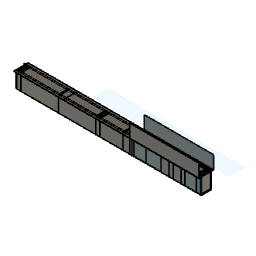
Final Bridge Assembly (Autodesk Fusion 360 design; units mm, degrees)
Autodesk Fusion 360 part; units mm, degrees
sketch "Sketch1" plane through (0, 0, 0) normal (0, 0, 1) x (1, 0, 0) in component "1: Left Top Flange "
  line L0 (20, 60) -> (364, 60)
  line L1 (364, 60) -> (364, -40)
  line L2 (364, -40) -> (20, -40)
  line L3 (20, -40) -> (20, 60)
  dimension "d1" = 344
  dimension "d2" = 100
  constraint horizontal L0
  constraint vertical L1
  constraint horizontal L2
  constraint vertical L3
  measures "d1" distance of L0.start L0.end
  measures "d2" distance of L0.start L2.end
extrude "Extrude1" add sketch "Sketch1" along normal blind 1.27 makes body 1 in component "1: Left Top Flange "
sketch "Sketch1 (2)" plane through (0, 0, 0) normal (0, 0, 1) x (1, 0, 0) in component "2: Left Top Flange"
  line L0 (109.7008, 156.6355) -> (917.5386, 156.6355)
  line L1 (917.5386, 156.6355) -> (917.5386, 56.6355)
  line L2 (917.5386, 56.6355) -> (109.7008, 56.6355)
  line L3 (109.7008, 56.6355) -> (109.7008, 156.6355)
  dimension "d5" = 807.8378
  dimension "d6" = 100
  constraint horizontal L0
  constraint vertical L1
  constraint horizontal L2
  constraint vertical L3
  measures "d5" distance of L0.start L0.end
  measures "d6" distance of L0.start L2.end
extrude "Extrude1'" add sketch "Sketch1 (2)" along normal blind 1.27 separate body makes body 2 in component "2: Left Top Flange"
sketch "Sketch1 (3)" plane through (0, 0, 0) normal (0, 0, 1) x (1, 0, 0) in component "3: Right Top Flange"
  line L0 (53.5373, 142.9301) -> (999.5373, 142.9301)
  line L1 (999.5373, 142.9301) -> (999.5373, 42.9301)
  line L2 (999.5373, 42.9301) -> (53.5373, 42.9301)
  line L3 (53.5373, 42.9301) -> (53.5373, 142.9301)
  line L4 (52.5635, 127.9301) -> (998.5635, 127.9301)
  line L5 (998.5635, 127.9301) -> (998.5635, 57.9301)
  line L6 (998.5635, 57.9301) -> (52.5635, 57.9301)
  line L7 (52.5635, 57.9301) -> (52.5635, 127.9301)
  dimension "d9" = 946
  dimension "d10" = 100
  dimension "d82" = 946
  dimension "d83" = 70
  dimension "d84" = 15
  constraint horizontal L0
  constraint vertical L1
  constraint horizontal L2
  constraint vertical L3
  constraint horizontal L4
  constraint vertical L5
  constraint horizontal L6
  constraint vertical L7
  measures "d9" distance of L0.start L0.end
  measures "d10" distance of L0.start L2.end
  measures "d82" distance of L4.start L4.end
  measures "d83" distance of L4.start L6.end
  measures "d84" distance of L0 L4
extrude "Extrude1''" add sketch "Sketch1 (3)" along normal blind 1.27 separate body contours L0 L1 L2 L3 L4 L5 L6 | L3 L4 L5 L6 makes body 3 in component "3: Right Top Flange"
sketch "Sketch1 (4)" plane through (0, 0, 0) normal (1, 0, 0) x (0, 1, 0)
  line L0 (84.0491, 337.799) -> (94.0491, 337.799)
  line L1 (94.0491, 337.799) -> (94.0491, 227.799)
  line L2 (94.0491, 227.799) -> (84.0491, 227.799)
  line L3 (84.0491, 227.799) -> (84.0491, 337.799)
  line L4 (145, 330) -> (136.27, 330)
  line L5 (94.0491, 282.799) -> (94.0491, 336.529)
  line L6 (94.0491, 336.529) -> (85.3191, 336.529)
  line L7 (85.3191, 336.529) -> (85.3191, 227.799)
  line L8 (85.3191, 227.799) -> (94.0491, 227.799)
  dimension "d13" = 10
  dimension "d14" = 110
  dimension "d15" = 8.73
  dimension "d18" = 8.73
  dimension "d73" = 1.27
  constraint horizontal L0
  constraint vertical L1
  constraint horizontal L2
  constraint vertical L3
  constraint horizontal L4
  constraint midpoint L1 L5.start
  constraint parallel L1 L5
  constraint perpendicular L5 L6
  constraint coincident L2 L7.end
  constraint perpendicular L2 L7
  measures "d13" distance of L0.start L0.end
  measures "d14" distance of L0.start L2.end
  measures "d15" distance of L4.start L4.end
  measures "d18" distance of L5.end L6.end
  measures "d73" distance of L0 L6
extrude "Extrude1'''" add sketch "Sketch1 (4)" along normal blind 807.8378 separate body contours L0 L1 L2 L3 L6 L7 makes body 4
copy_body "Body->Comp1" bodies 4 removing the originals makes body 5 in component "4: Left Web"
sketch "Sketch1 (5)" plane through (0, 0, 0) normal (1, 0, 0) x (0, 1, 0) in component "6: Right Web"
  line L0 (125, 150) -> (135, 150)
  line L1 (135, 150) -> (135, 40)
  line L2 (135, 40) -> (125, 40)
  line L3 (125, 40) -> (125, 150)
  line L4 (135, 148.73) -> (126.27, 148.73)
  line L5 (126.27, 148.73) -> (126.27, 41.27)
  line L6 (126.27, 41.27) -> (135, 41.27)
  dimension "d21" = 10
  dimension "d22" = 110
  dimension "d23" = 1.27
  dimension "d24" = 8.73
  dimension "d25" = 107.46
  constraint horizontal L0
  constraint vertical L1
  constraint horizontal L2
  constraint vertical L3
  constraint coincident L1 L4.start
  constraint perpendicular L1 L4
  constraint perpendicular L4 L5
  constraint coincident L1 L6.end
  constraint perpendicular L1 L6
  measures "d21" distance of L0.start L0.end
  measures "d22" distance of L0.start L2.end
  measures "d23" distance of L0 L4
  measures "d24" distance of L4.start L4.end
  measures "d25" distance of L4.end L5.end
sketch "Sketch2" plane through (0, 0, 0) normal (1, 0, 0) x (0, 1, 0) in component "6: Right Web"
  line L0 (75, 175) -> (85, 175)
  line L1 (85, 175) -> (85, 65)
  line L2 (85, 65) -> (75, 65)
  line L3 (75, 65) -> (75, 175)
  line L4 (85, 173.73) -> (76.27, 173.73)
  line L5 (76.27, 173.73) -> (76.27, 66.27)
  line L6 (76.27, 66.27) -> (85, 66.27)
  line L7 (85, 66.27) -> (85, 173.73)
  dimension "d28" = 10
  dimension "d29" = 110
  dimension "d30" = 8.73
  dimension "d31" = 107.46
  dimension "d32" = 1.27
  constraint horizontal L0
  constraint vertical L1
  constraint horizontal L2
  constraint vertical L3
  constraint horizontal L4
  constraint vertical L5
  constraint horizontal L6
  constraint vertical L7
  constraint coincident L1 L4.start
  measures "d28" distance of L0.start L0.end
  measures "d29" distance of L0.start L2.end
  measures "d30" distance of L4.start L4.end
  measures "d31" distance of L4.start L6.end
  measures "d32" distance of L0 L4
extrude "Extrude1''''" add sketch "Sketch2" along normal blind 482.1622 separate body contours L0 L1 L2 L3 L4 L5 L6 makes body 6 in component "6: Right Web"
sketch "Sketch1 (6)" plane through (0, 0, 1.27) normal (0, 0, 1) x (-1, 0, 0) in component "5: Bottom Flange"
  line L0 (-16.1175, -67.934) -> (-360.1175, -67.934)
  line L1 (-360.1175, -67.934) -> (-360.1175, -167.934)
  line L2 (-360.1175, -167.934) -> (-16.1175, -167.934)
  line L3 (-16.1175, -167.934) -> (-16.1175, -67.934)
  line L4 (200, -300) -> (-282.1622, -300)
  line L5 (-282.1622, -300) -> (-282.1622, -230)
  line L6 (-282.1622, -230) -> (200, -230)
  line L7 (200, -230) -> (200, -300)
  dimension "d35" = 482.1622
  dimension "d36" = 70
  constraint horizontal L4
  constraint vertical L5
  constraint horizontal L6
  constraint vertical L7
  measures "d35" distance of L4.start L4.end
  measures "d36" distance of L4.start L6.end
extrude "Extrude1'''''" add sketch "Sketch1 (6)" along normal blind 1.27 separate body contours L4 L5 L6 L7 makes body 7 in component "5: Bottom Flange"
sketch "Sketch1 (7)" plane through (0, 0, 0) normal (0, 1, 0) x (1, 0, 0) in component "7: Diaphragm"
  line L0 (40, -120) -> (50, -120)
  line L1 (50, -120) -> (50, -10)
  line L2 (50, -10) -> (40, -10)
  line L3 (40, -10) -> (40, -120)
  line L4 (41.27, -118.73) -> (50, -118.73)
  line L5 (50, -118.73) -> (50, -11.27)
  line L6 (50, -11.27) -> (41.27, -11.27)
  line L7 (41.27, -11.27) -> (41.27, -118.73)
  dimension "d39" = 10
  dimension "d40" = 110
  dimension "d41" = 8.73
  dimension "d42" = 107.46
  dimension "d43" = 1.27
  dimension "d44" = 1.27
  constraint horizontal L0
  constraint vertical L1
  constraint horizontal L2
  constraint vertical L3
  constraint horizontal L4
  constraint vertical L5
  constraint horizontal L6
  constraint vertical L7
  measures "d39" distance of L0.start L0.end
  measures "d40" distance of L0.start L2.end
  measures "d41" distance of L4.start L4.end
  measures "d42" distance of L4.start L6.end
  measures "d43" distance of L0 L4
  measures "d44" distance of L3 L7
extrude "Extrude1''''''" add sketch "Sketch1 (7)" along normal blind 70 separate body contours L0 L1 L2 L3 L4 L6 L7 makes body 8 in component "7: Diaphragm"
sketch "Sketch1 (8)" plane through (0, 0, 0) normal (0, 1, 0) x (1, 0, 0) in component "8: B Support"
  line L0 (26.8308, -313.1961) -> (166.8308, -313.1961)
  line L1 (166.8308, -313.1961) -> (166.8308, -203.1961)
  line L2 (166.8308, -203.1961) -> (26.8308, -203.1961)
  line L3 (26.8308, -203.1961) -> (26.8308, -313.1961)
  dimension "d47" = 140
  dimension "d48" = 110
  constraint horizontal L0
  constraint vertical L1
  constraint horizontal L2
  constraint vertical L3
  measures "d47" distance of L0.start L0.end
  measures "d48" distance of L0.start L2.end
extrude "Extrude1'''''''" add sketch "Sketch1 (8)" along normal blind 1.27 separate body makes body 9 in component "8: B Support"
sketch "Sketch1 (9)" plane through (0, 0, 0) normal (1, 0, 0) x (0, 1, 0) in component "9: Top Flap"
  line L0 (150, 200) -> (160, 200)
  line L1 (160, 200) -> (160, 107)
  line L2 (160, 107) -> (150, 107)
  line L3 (150, 107) -> (150, 200)
  line L4 (160, 200) -> (151.27, 200)
  line L5 (151.27, 200) -> (151.27, 108.27)
  line L6 (151.27, 108.27) -> (160, 108.27)
  line L7 (160, 108.27) -> (160, 200)
  dimension "d51" = 10
  dimension "d52" = 93
  dimension "d53" = 8.73
  dimension "d54" = 91.73
  constraint horizontal L0
  constraint vertical L1
  constraint horizontal L2
  constraint vertical L3
  constraint horizontal L4
  constraint vertical L5
  constraint horizontal L6
  constraint vertical L7
  measures "d51" distance of L0.start L0.end
  measures "d52" distance of L0.start L2.end
  measures "d53" distance of L0.end L4.end
  measures "d54" distance of L0.end L6.end
extrude "Extrude1''''''''" add sketch "Sketch1 (9)" along normal blind 482.1622 separate body contours L0 L1 L2 L3 L5 L6 makes body 10 in component "9: Top Flap"
sketch "Sketch2 (2)" plane through (0, -8.9412, 144.9104) normal (0, 0, -1) x (1, 0, 0)
  line L0 (669.5376, -297.9716) -> (-276.4624, -297.9716)
  line L1 (-276.4624, -297.9716) -> (-276.4624, -397.9716)
  line L2 (-276.4624, -397.9716) -> (669.5376, -397.9716)
  line L3 (669.5376, -397.9716) -> (669.5376, -297.9716)
sketch "Sketch3" plane through (0, 0, 0) normal (0, 0, 1) x (1, 0, 0)
sketch "Sketch1 (10)" plane through (0, 0, 0) normal (0, 1, 0) x (1, 0, 0) in component "Left Diaphragms"
  line L0 (-832.5114, -19.9115) -> (-822.5114, -19.9115)
  line L1 (-822.5114, -19.9115) -> (-822.5114, 91.3585)
  line L2 (-822.5114, 91.3585) -> (-832.5114, 91.3585)
  line L3 (-832.5114, 91.3585) -> (-832.5114, -19.9115)
  line L4 (-822.5114, 91.3585) -> (-831.2414, 91.3585)
  line L5 (-831.2414, 91.3585) -> (-831.2414, -18.6415)
  line L6 (-831.2414, -18.6415) -> (-822.5114, -18.6415)
  line L7 (-822.5114, -18.6415) -> (-822.5114, 91.3585)
  dimension "d155" = 10
  dimension "d156" = 111.27
  dimension "d157" = 8.73
  dimension "d158" = 110
  constraint horizontal L0
  constraint vertical L1
  constraint horizontal L2
  constraint vertical L3
  constraint horizontal L4
  constraint vertical L5
  constraint horizontal L6
  constraint vertical L7
  measures "d155" distance of L0.start L0.end
  measures "d156" distance of L0.start L2.end
  measures "d157" distance of L1.end L4.end
  measures "d158" distance of L1.end L6.end
extrude "Extrude1'''''''''" add sketch "Sketch1 (10)" along normal blind 70 separate body contours L0 L1 L2 L3 L5 L6 makes body 11 in component "Left Diaphragms"
copy_body "CopyPasteBodies1" bodies 11 makes body 12 in component "Left Diaphragms"
copy_body "CopyPasteBodies2" bodies 11 makes body 13 in component "Left Diaphragms"
copy_body "CopyPasteBodies3" bodies 11 12 13 makes body 14 makes body 15 makes body 16 in component "Left Diaphragms"
sketch "Sketch4" plane through (0, 307.7518, 0) normal (0, -1, 0) x (1, 0, 0)
  line L0 (-837.6631, 18.8471) -> (-837.6631, -91.1529)
  line L1 (-837.6631, -91.1529) -> (-29.8253, -91.1529)
  line L2 (-29.8253, -91.1529) -> (-29.8253, 18.8471)
  line L3 (-29.8253, 18.8471) -> (-837.6631, 18.8471)
  line L4 (-44.0073, 18.8471) -> (-14.0073, 18.8471)
  line L5 (-14.0073, 18.8471) -> (-14.0073, -91.1529)
  line L6 (-14.0073, -91.1529) -> (-44.0073, -91.1529)
  line L7 (-44.0073, -91.1529) -> (-44.0073, 18.8471)
  dimension "d193" = 30
  dimension "d194" = 110
  constraint horizontal L4
  constraint vertical L5
  constraint horizontal L6
  constraint vertical L7
  constraint coincident L3 L4.start
  measures "d193" distance of L4.start L4.end
  measures "d194" distance of L4.start L6.end
extrude "Extrude2" add sketch "Sketch4" along normal blind 1.27 contours L1 L2 L3 L4 L6 L7 | L2 L4 L5 L6 sketch seen with x (1, 0, 0) y (0, 1, 0) z (0, 0, 1) at (947.3639, -236.1163, -18.8471) bodies 2 in component "2: Left Top Flange"
sketch "Sketch5" plane through (0, 306.4818, 0) normal (0, -1, 0) x (1, 0, 0)
  line L0 (-44.0072, -91.1529) -> (-14.0072, -91.1529)
  line L1 (-14.0072, -91.1529) -> (-14.0072, 18.8471)
  line L2 (-14.0072, 18.8471) -> (-29.8253, 18.8471)
  line L3 (-29.8253, 18.8471) -> (-44.0072, 18.8471)
  line L4 (-44.0072, 18.8471) -> (-44.0072, -91.1529)
sketch "Sketch6" plane through (0, 377.7518, 0) normal (0, 1, 0) x (-1, 0, 0)
  line L0 (29.8253, 18.8471) -> (29.8253, -91.1529)
  line L1 (29.8253, -91.1529) -> (837.6631, -91.1529)
  line L2 (837.6631, -91.1529) -> (837.6631, 18.8471)
  line L3 (837.6631, 18.8471) -> (29.8253, 18.8471)
  line L4 (29.8253, 18.8471) -> (44.8253, 18.8471)
  line L5 (44.8253, 18.8471) -> (44.8253, -91.1529)
  line L6 (44.8253, -91.1529) -> (29.8253, -91.1529)
  line L7 (29.8253, -91.1529) -> (29.8253, 18.8471)
  line L8 (29.8253, 18.8471) -> (14.8253, 18.8471)
  line L9 (14.8253, 18.8471) -> (14.8253, -91.1529)
  line L10 (14.8253, -91.1529) -> (29.8253, -91.1529)
  line L11 (29.8253, -91.1529) -> (29.8253, 18.8471)
  dimension "d197" = 15
  dimension "d198" = 110
  dimension "d199" = 110
  constraint horizontal L4
  constraint vertical L5
  constraint horizontal L6
  constraint vertical L7
  constraint coincident L0.start L3.end
  constraint horizontal L8
  constraint vertical L9
  constraint horizontal L10
  constraint vertical L11
  measures "d197" distance of L0.start L4.end
  measures "d198" distance of L0.start L0.end
  measures "d199" distance of L0.start L0.end
extrude "Extrude3" add sketch "Sketch6" along normal blind 1.27 contours L0 L1 L3 L4 L5 L6 L7 L11 | L0 L7 L8 L9 L10 L11 sketch seen with x (1, 0, 0) y (0, 1, 0) z (0, 0, 1) at (947.3639, -236.1163, -18.8471) bodies 2 in component "2: Left Top Flange"
delete_face "DeleteFace1" 1 faces at (918.084, 70.3655, -73.3333) on bodies 2 in component "2: Left Top Flange"
sketch "Sketch7" plane through (0, 307.7518, 0) normal (0, -1, 0) x (1, 0, 0)
  line L0 (-29.8253, 20.1171) -> (-29.8253, -89.8829)
  line L1 (-29.8253, -89.8829) -> (452.3369, -89.8829)
  line L2 (452.3369, -89.8829) -> (452.3369, 20.1171)
  line L3 (452.3369, 20.1171) -> (-29.8253, 20.1171)
extrude "Extrude4" add sketch "Sketch5" along normal blind 1.27 sketch seen with x (1, 0, 0) y (0, 1, 0) z (0, 0, 1) at (947.3639, -236.1163, -18.8471) bodies 2 in component "2: Left Top Flange"
delete_face "DeleteFace2" 1 faces at (918.084, 69.0955, -73.3333) on bodies 2 in component "2: Left Top Flange"
sketch "Sketch8" plane through (0, 307.7518, 0) normal (0, -1, 0) x (1, 0, 0)
  line L0 (-837.6631, 18.8471) -> (-837.6631, -91.1529)
  line L1 (-837.6631, -91.1529) -> (-29.8253, -91.1529)
  line L2 (-29.8253, -91.1529) -> (-29.8253, 18.8471)
  line L3 (-29.8253, 18.8471) -> (-837.6631, 18.8471)
  line L4 (-29.8253, 18.8471) -> (-14.8253, 18.8471)
  line L5 (-14.8253, 18.8471) -> (-14.8253, -91.1529)
  line L6 (-14.8253, -91.1529) -> (-29.8253, -91.1529)
  line L7 (-29.8253, -91.1529) -> (-29.8253, 18.8471)
  line L8 (-29.8253, 18.8471) -> (-44.8253, 18.8471)
  line L9 (-44.8253, 18.8471) -> (-44.8253, -91.1529)
  line L10 (-44.8253, -91.1529) -> (-29.8253, -91.1529)
  line L11 (-29.8253, -91.1529) -> (-29.8253, 18.8471)
  dimension "d208" = 15
  dimension "d209" = 110
  dimension "d210" = 110
  constraint horizontal L4
  constraint vertical L5
  constraint horizontal L6
  constraint vertical L7
  constraint coincident L2.end L3.start
  constraint horizontal L8
  constraint vertical L9
  constraint horizontal L10
  constraint vertical L11
  measures "d208" distance of L2.end L4.end
  measures "d209" distance of L2.end L1.end
  measures "d210" distance of L2.end L1.end
extrude "Extrude2'" add sketch "Sketch8" along normal blind 1.27 contours L1 L2 L3 L7 L8 L9 L10 L11 | L2 L4 L5 L6 L7 L11 sketch seen with x (1, 0, 0) y (0, 1, 0) z (0, 0, 1) at (837.6631, -223.7027, 318.952) bodies 5 in component "4: Left Web"
component "1: Left Top Flange " placed x (1, 0, 0) y (0, 1, 0) z (0, 0, 1) at (-857.6631, 332.7518, 20.1171)
component "2: Left Top Flange" placed x (1, 0, 0) y (0, 1, 0) z (0, 0, 1) at (-947.3639, 236.1163, 18.8471)
component "3: Right Top Flange" placed x (1, 0, 0) y (0, 1, 0) z (0, 0, 1) at (-547.2004, 249.8217, 20.1171)
component "4: Left Web" placed x (1, 0, 0) y (0, 1, 0) z (0, 0, 1) at (-837.6631, 223.7027, -318.952)
component "6: Right Web" placed x (1, 0, 0) y (0, 1, 0) z (0, 0, 1) at (-29.8253, 232.7518, -154.8829)
component "5: Bottom Flange" placed x (1, 0, 0) y (0, 1, 0) z (0, 0, 1) at (170.1747, 77.7518, -92.4229)
component "8: B Support" placed x (1, 0, 0) y (0, 1, 0) z (0, 0, 1) at (145.5061, 306.4818, -293.0791)
component "9: Top Flap" placed x (1, 0, 0) y (0, 1, 0) z (0, 0, 1) at (-29.8253, 141.4818, -88.1529)
component "4: Left Web" placed x (-1, 0, 0) y (0, -1, 0) z (0, 0, 1) at (-29.8253, 461.8009, -318.952)
component "6: Right Web" placed x (-1, 0, 0) y (0, -1, 0) z (0, 0, 1) at (452.3369, 452.7518, -154.8829)
component "9: Top Flap" placed x (-1, 0, 0) y (0, -1, 0) z (0, 0, 1) at (452.3369, 544.0218, -88.1529)
component "8: B Support" placed x (1, 0, 0) y (0, 1, 0) z (0, 0, 1) at (145.5061, 377.7518, -293.0791)
component "7: Diaphragm" placed x (1, 0, 0) y (0, 1, 0) z (0, 0, 1) at (27.3369, 307.7518, -99.8829)
component "7: Diaphragm" placed x (1, 0, 0) y (0, 1, 0) z (0, 0, 1) at (377.3369, 307.7518, -99.8829)
component "7: Diaphragm" placed x (-1, 0, 0) y (0, -1, 0) z (0, 0, 1) at (297.3369, 377.7518, -99.8829)
component "7: Diaphragm" placed x (-1, 0, 0) y (0, -1, 0) z (0, 0, 1) at (487.3369, 377.7518, -99.8829)
component "7: Diaphragm" placed x (1, 0, 0) y (0, 1, 0) z (0, 0, 1) at (187.3369, 307.7518, -99.8829)
component "7: Diaphragm" placed x (1, 0, 0) y (0, 1, 0) z (0, 0, 1) at (297.3369, 307.7518, -99.8829)
component "7: Diaphragm" placed x (1, 0, 0) y (0, 1, 0) z (0, 0, 1) at (187.3369, 307.7518, -99.8829)
component "Left Diaphragms" placed x (1, 0, 0) y (0, 1, 0) z (0, 0, 1) at (-0.1517, 307.7518, 0.2055)
component "Left Diaphragms" placed x (-1, 0, 0) y (0, -1, 0) z (0, 0, 1) at (-1635.1745, 377.7518, 0.2055)
component "Left Diaphragms" placed x (1, 0, 0) y (0, 1, 0) z (0, 0, 1) at (289.8483, 307.7518, 0.2055)
component "Left Diaphragms" placed x (-1, 0, 0) y (0, -1, 0) z (0, 0, 1) at (-1085.1745, 377.7518, 0.2055)
component "Left Diaphragms" placed x (1, 0, 0) y (0, 1, 0) z (0, 0, 1) at (549.8483, 307.7518, 0.2055)
component "Left Diaphragms" placed x (1, 0, 0) y (0, 1, 0) z (0, 0, 1) at (739.8483, 307.7518, 0.2055)
component "7: Diaphragm" placed x (-1, 0, 0) y (0, -1, 0) z (0, 0, 1) at (297.3369, 377.7518, -99.8829)
